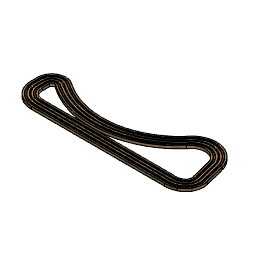
mdf_track (Autodesk Fusion 360 design; units mm, degrees)
part number: 2026-04-03-14-52-22-321
Autodesk Fusion 360 part; units mm, degrees
note: some values were not read from the file. Chosen so that the rebuilt part matches the saved one: which bodies a step acts on.
sketch "Sketch1" plane through (0, 0, 0) normal (0, 0, 1) x (1, 0, 0)
  line L0 (0, 0) -> (1270, 0) construction
  line L1 (158.75, 0) -> (1111.25, 0)
  arc A0 (87.8541, 15.7546) -> (158.75, 0) centre (158.75, 167.3931) ccw
  arc A1 (1111.25, 0) -> (1185.6577, 16.6251) centre (1111.25, 174.8234) ccw
  line L2 (0, 153.8111) -> (0, 203.2)
  arc A2 (159.5434, 286.6573) -> (0, 203.2) centre (101.6, 203.2) ccw
  line L3 (1254.8125, 162.3499) -> (1219.2, 304.8)
  arc A3 (1219.2, 304.8) -> (891.9874, 360.3055) centre (1043.432, 260.858) ccw
  arc A4 (159.5434, 286.6573) -> (185.665, 269.3614) centre (565.1474, 870.8583) ccw
  arc A5 (185.665, 269.3614) -> (891.9874, 360.3055) centre (483.8297, 741.9661) ccw
  arc A6 (1185.6577, 16.6251) -> (1254.8125, 162.3499) centre (1131.6044, 131.5478) ccw
  arc A7 (0, 153.8111) -> (87.8541, 15.7546) centre (152.4, 153.8111) ccw
  dimension "d1" = 1270
  dimension "d2" = 952.5
  dimension "d3" = 158.75
  dimension "d4" = 711.2
  dimension "d5" = 558.8
  dimension "d6" = 127
  dimension "d7" = 152.4
  constraint coincident L0.start origin
  constraint horizontal L0
  constraint coincident L0 L1.start
  constraint coincident L0 L1.end
  constraint tangent L0 A0
  constraint tangent L0 A1
  constraint vertical L2
  constraint tangent L2 A2
  constraint tangent L3 A3
  constraint tangent A2 A4
  constraint tangent A4 A5
  constraint tangent A1 A6
  constraint tangent L3 A6
  constraint tangent A0 A7
  constraint tangent L2 A7
  measures "d1" distance of L0.start L0.end
  measures "d2" distance of L1.start L1.end
  measures "d3" distance of L0.start L1.start
  measures "d4" radius of A4
  measures "d5" radius of A5
  measures "d6" radius of A6
  measures "d7" radius of A7
extrude "Extrude1" add sketch "Sketch1" along normal blind 19.05 makes body 1
sketch "Sketch2" plane through (0, 0, 19.05) normal (0, 0, 1) x (-1, 0, 0)
  arc A0 (-159.5434, -286.6573) -> (0, -203.2) centre (-101.6, -203.2) ccw
  line L0 (0, -203.2) -> (0, -153.8111)
  arc A1 (0, -153.8111) -> (-87.8541, -15.7546) centre (-152.4, -153.8111) ccw
  arc A2 (-87.8541, -15.7546) -> (-158.75, 0) centre (-158.75, -167.3931) ccw
  line L1 (-158.75, 0) -> (-1111.25, 0)
  arc A3 (-1111.25, 0) -> (-1185.6577, -16.6251) centre (-1111.25, -174.8234) ccw
  arc A4 (-1185.6577, -16.6251) -> (-1254.8125, -162.3499) centre (-1131.6044, -131.5478) ccw
  line L2 (-1254.8125, -162.3499) -> (-1219.2, -304.8)
  arc A5 (-1219.2, -304.8) -> (-891.9874, -360.3055) centre (-1043.432, -260.858) ccw
  arc A6 (-185.665, -269.3614) -> (-891.9874, -360.3055) centre (-483.8297, -741.9661) ccw
  arc A7 (-159.5434, -286.6573) -> (-185.665, -269.3614) centre (-565.1474, -870.8583) ccw
  arc A8 (-1139.1147, -284.7787) -> (-957.9655, -310.0806) centre (-1043.432, -260.858) ccw
  arc A9 (-141.618, -199.5448) -> (-957.9655, -310.0806) centre (-483.8297, -741.9661) ccw
  arc A10 (-112.4644, -218.8482) -> (-141.618, -199.5448) centre (-565.1474, -870.8583) ccw
  arc A11 (-112.4644, -218.8482) -> (-82.55, -203.2) centre (-101.6, -203.2) ccw
  line L3 (-82.55, -203.2) -> (-82.55, -153.8111)
  arc A12 (-82.55, -153.8111) -> (-122.8165, -90.5352) centre (-152.4, -153.8111) ccw
  arc A13 (-122.8165, -90.5352) -> (-158.75, -82.55) centre (-158.75, -167.3931) ccw
  line L4 (-158.75, -82.55) -> (-1111.25, -82.55)
  arc A14 (-1111.25, -82.55) -> (-1150.5231, -91.3249) centre (-1111.25, -174.8234) ccw
  arc A15 (-1150.5231, -91.3249) -> (-1174.7273, -142.3285) centre (-1131.6044, -131.5478) ccw
  line L5 (-1174.7273, -142.3285) -> (-1139.1147, -284.7787)
  arc A16 (-1206.8792, -301.7198) -> (-902.0233, -352.4454) centre (-1043.432, -260.858) ccw
  arc A17 (-178.8886, -258.6204) -> (-902.0233, -352.4454) centre (-483.8297, -741.9661) ccw
  arc A18 (-152.3005, -276.2251) -> (-178.8886, -258.6204) centre (-565.1474, -870.8583) ccw
  arc A19 (-152.3005, -276.2251) -> (-12.7, -203.2) centre (-101.6, -203.2) ccw
  line L6 (-12.7, -203.2) -> (-12.7, -153.8111)
  arc A20 (-12.7, -153.8111) -> (-93.2329, -27.2593) centre (-152.4, -153.8111) ccw
  arc A21 (-93.2329, -27.2593) -> (-158.75, -12.7) centre (-158.75, -167.3931) ccw
  line L7 (-158.75, -12.7) -> (-1111.25, -12.7)
  arc A22 (-1111.25, -12.7) -> (-1180.2524, -28.1173) centre (-1111.25, -174.8234) ccw
  arc A23 (-1180.2524, -28.1173) -> (-1242.4917, -159.2696) centre (-1131.6044, -131.5478) ccw
  line L8 (-1242.4917, -159.2696) -> (-1206.8792, -301.7198)
  arc A24 (-1196.2076, -299.0519) -> (-910.7445, -345.6708) centre (-1043.432, -260.858) ccw
  arc A25 (-173.0192, -249.3171) -> (-910.7445, -345.6708) centre (-483.8297, -741.9661) ccw
  arc A26 (-146.0271, -267.1894) -> (-173.0192, -249.3171) centre (-565.1474, -870.8583) ccw
  arc A27 (-146.0271, -267.1894) -> (-23.7, -203.2) centre (-101.6, -203.2) ccw
  line L9 (-23.7, -203.2) -> (-23.7, -153.8111)
  arc A28 (-23.7, -153.8111) -> (-97.8918, -37.2241) centre (-152.4, -153.8111) ccw
  arc A29 (-97.8918, -37.2241) -> (-158.75, -23.7) centre (-158.75, -167.3931) ccw
  line L10 (-158.75, -23.7) -> (-1111.25, -23.7)
  arc A30 (-1111.25, -23.7) -> (-1175.5706, -38.0713) centre (-1111.25, -174.8234) ccw
  arc A31 (-1175.5706, -38.0713) -> (-1231.8201, -156.6018) centre (-1131.6044, -131.5478) ccw
  line L11 (-1231.8201, -156.6018) -> (-1196.2076, -299.0519)
  arc A32 (-1151.4355, -287.8589) -> (-947.6802, -317.6507) centre (-1043.432, -260.858) ccw
  arc A33 (-148.3944, -210.2858) -> (-947.6802, -317.6507) centre (-483.8297, -741.9661) ccw
  arc A34 (-119.7073, -229.2804) -> (-148.3944, -210.2858) centre (-565.1474, -870.8583) ccw
  arc A35 (-119.7073, -229.2804) -> (-69.85, -203.2) centre (-101.6, -203.2) ccw
  line L12 (-69.85, -203.2) -> (-69.85, -153.8111)
  arc A36 (-69.85, -153.8111) -> (-117.4376, -79.0305) centre (-152.4, -153.8111) ccw
  arc A37 (-117.4376, -79.0305) -> (-158.75, -69.85) centre (-158.75, -167.3931) ccw
  line L13 (-158.75, -69.85) -> (-1111.25, -69.85)
  arc A38 (-1111.25, -69.85) -> (-1155.9284, -79.8326) centre (-1111.25, -174.8234) ccw
  arc A39 (-1155.9284, -79.8326) -> (-1187.0481, -145.4087) centre (-1131.6044, -131.5478) ccw
  line L14 (-1187.0481, -145.4087) -> (-1151.4355, -287.8589)
  arc A40 (-1162.1053, -290.5263) -> (-938.8203, -324.2613) centre (-1043.432, -260.858) ccw
  arc A41 (-154.2629, -219.5875) -> (-938.8203, -324.2613) centre (-483.8297, -741.9661) ccw
  arc A42 (-125.9797, -238.3147) -> (-154.2629, -219.5875) centre (-565.1474, -870.8583) ccw
  arc A43 (-125.9797, -238.3147) -> (-58.8518, -203.2) centre (-101.6, -203.2) ccw
  line L15 (-58.8518, -203.2) -> (-58.8518, -153.8111)
  arc A44 (-58.8518, -153.8111) -> (-112.7796, -69.0674) centre (-152.4, -153.8111) ccw
  arc A45 (-112.7796, -69.0674) -> (-158.75, -58.8518) centre (-158.75, -167.3931) ccw
  line L16 (-158.75, -58.8518) -> (-1111.25, -58.8518)
  arc A46 (-1111.25, -58.8518) -> (-1160.6094, -69.8803) centre (-1111.25, -174.8234) ccw
  arc A47 (-1160.6094, -69.8803) -> (-1197.7179, -148.0762) centre (-1131.6044, -131.5478) ccw
  line L17 (-1197.7179, -148.0762) -> (-1162.1053, -290.5263)
  arc A48 (-1176.0771, -294.0193) -> (-927.2764, -332.985) centre (-1043.432, -260.858) ccw
  arc A49 (-161.9474, -231.7678) -> (-927.2764, -332.985) centre (-483.8297, -741.9661) ccw
  arc A50 (-134.1932, -250.1447) -> (-161.9474, -231.7678) centre (-565.1474, -870.8583) ccw
  arc A51 (-134.1932, -250.1447) -> (-44.45, -203.2) centre (-101.6, -203.2) ccw
  line L18 (-44.45, -203.2) -> (-44.45, -153.8111)
  arc A52 (-44.45, -153.8111) -> (-106.68, -56.0211) centre (-152.4, -153.8111) ccw
  arc A53 (-106.68, -56.0211) -> (-158.75, -44.45) centre (-158.75, -167.3931) ccw
  line L19 (-158.75, -44.45) -> (-1111.25, -44.45)
  arc A54 (-1111.25, -44.45) -> (-1166.739, -56.848) centre (-1111.25, -174.8234) ccw
  arc A55 (-1166.739, -56.848) -> (-1211.6897, -151.5691) centre (-1131.6044, -131.5478) ccw
  line L20 (-1211.6897, -151.5691) -> (-1176.0771, -294.0193)
  arc A56 (-1182.2376, -295.5594) -> (-922.2054, -336.8533) centre (-1043.432, -260.858) ccw
  arc A57 (-165.3356, -237.1383) -> (-922.2054, -336.8533) centre (-483.8297, -741.9661) ccw
  arc A58 (-137.8146, -255.3608) -> (-165.3356, -237.1383) centre (-565.1474, -870.8583) ccw
  arc A59 (-137.8146, -255.3608) -> (-38.1, -203.2) centre (-101.6, -203.2) ccw
  line L21 (-38.1, -203.2) -> (-38.1, -153.8111)
  arc A60 (-38.1, -153.8111) -> (-103.9906, -50.2688) centre (-152.4, -153.8111) ccw
  arc A61 (-103.9906, -50.2688) -> (-158.75, -38.1) centre (-158.75, -167.3931) ccw
  line L22 (-158.75, -38.1) -> (-1111.25, -38.1)
  arc A62 (-1111.25, -38.1) -> (-1169.4417, -51.1019) centre (-1111.25, -174.8234) ccw
  arc A63 (-1169.4417, -51.1019) -> (-1217.8501, -153.1092) centre (-1131.6044, -131.5478) ccw
  line L23 (-1217.8501, -153.1092) -> (-1182.2376, -295.5594)
  dimension "d10" = 82.55
  dimension "d11" = 12.7
  dimension "d12" = 11
  dimension "d13" = -12.7
  dimension "d14" = -10.9982
  dimension "d19" = -38.1
  dimension "d20" = 38.1
extrude "Extrude2" cut sketch "Sketch2" against normal blind 50.8 contours A8 A9 A10 A11 L3 A12 A13 L4 A14 A15 L5 | A56 A57 A58 A59 L21 A60 A61 L22 A62 A63 L23 bodies 1 makes body 2 at (476.25, 25.4, 19.05)
extrude "Extrude3" cut sketch "Sketch2" against normal blind 2.54 contours A16 A17 A18 A19 L6 A20 A21 L7 A22 A23 L8 | A40 A41 A42 A43 L15 A44 A45 L16 A46 A47 L17 bodies 1 2
equation "d2 = d1 * 3 / 4"
equation "d3 = d1 * 1 / 8"
